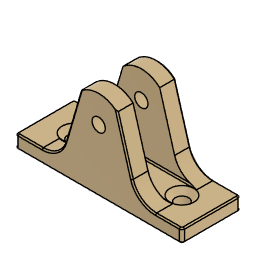
Trava toldo Regal v2 (Autodesk Fusion 360 design; units mm, degrees)
Autodesk Fusion 360 part; units mm, degrees
sketch "Sketch1" plane through (0, 0, 0) normal (0, 1, 0) x (1, 0, 0)
  line L0 (0, 0) -> (62.5, 0)
  line L1 (62.5, 0) -> (62.5, -5)
  line L2 (62.5, -5) -> (52.5, -5)
  arc A0 (52.5, -5) -> (43.75, -11.5668) centre (52.5, -14.1129) ccw
  line L3 (43.75, -11.5668) -> (38.15, -30.812)
  arc A1 (24.35, -30.812) -> (38.15, -30.812) centre (31.25, -23.3) ccw
  line L4 (24.35, -30.812) -> (18.75, -11.5668)
  arc A2 (18.75, -11.5668) -> (10, -5) centre (10, -14.1129) ccw
  line L5 (10, -5) -> (0, -5)
  line L6 (0, -5) -> (0, 0)
  circle A3 centre (31.25, -23.3) radius 2.5
  line L7 (24.35, -30.812) -> (38.15, -30.812) construction
  line L8 (31.25, -33.5) -> (31.25, -23.3) construction
  line L9 (10, -5) -> (52.5, -5)
  dimension "d1" = 13.8
  dimension "d2" = 7.7
  dimension "d3" = 5
  dimension "d5" = 5
  dimension "d8" = 62.5
  dimension "d29" = 33.5
  dimension "d30" = 25
  dimension "d31" = 10
  constraint coincident L0.start L6.end
  constraint horizontal L0
  constraint perpendicular L0 L1
  constraint perpendicular L1 L2
  constraint tangent L2 A0
  constraint tangent L4 A2
  constraint horizontal L5
  constraint perpendicular L0 L6
  constraint concentric A1 A3
  constraint horizontal L7
  constraint equal L3 L4
  constraint tangent A2 L5
  constraint tangent A0 L3
  constraint midpoint A1 L8.start
  constraint coincident A1.centre A3.centre
  constraint equal L2 L5
  constraint equal L1 L6
  constraint equal A0 A2
  measures "d1" distance of L3.end A1.start
  measures "d2" distance of A1 A3
  measures "d3" diameter of A3
  measures "d5" distance of L5.end L0.start
  measures "d8" distance of L0.start L0.end
  measures "d29" distance of L0 L8.start
  measures "d30" distance of A0.end L4.end
  measures "d31" distance of A2.end L5.end
extrude "Extrude1" add sketch "Sketch1" along normal blind 6
extrude "Extrude2" add sketch "Sketch1" against normal blind 10 contours L0 L1 L2 L5 L6 L9
extrude "Extrude3" add 1 faces at (31.3123, 6, 14.6469) along direction (0, -1, 0) blind 6 from surface at 16
fillet "Fillet1" radius 1 4 edges at (0, -16, 2.5) (62.5, -16, 2.5) (62.5, 6, 2.5) (0, 6, 2.5)
sketch "Sketch2" plane through (0, 0, 0) normal (0, 0, -1) x (1, 0, 0)
  arc A0 (0, -5) -> (1, -6) centre (1, -5) ccw
  line L0 (1, -6) -> (61.5, -6)
  arc A1 (61.5, -6) -> (62.5, -5) centre (61.5, -5) ccw
  line L1 (62.5, -5) -> (62.5, 15)
  arc A2 (62.5, 15) -> (61.5, 16) centre (61.5, 15) ccw
  line L2 (61.5, 16) -> (1, 16)
  arc A3 (1, 16) -> (0, 15) centre (1, 15) ccw
  line L3 (0, 15) -> (0, -5)
  line L4 (0, 5) -> (62.5, 5) construction
  circle A4 centre (11, 5) radius 2.5
  circle A5 centre (51.5, 5) radius 2.5
  line L5 (31.25, 5) -> (31.25, 16) construction
  dimension "d20" = 40.5
  dimension "d21" = 5
  constraint midpoint L3 L4.start
  constraint midpoint L1 L4.end
  constraint coincident L4 A4.centre
  constraint coincident L4 A5.centre
  constraint equal A4 A5
  constraint midpoint L4 L5.start
  constraint midpoint L2 L5.end
  constraint symmetric A4 A5 L5
  measures "d20" distance of A4.centre A5.centre
  measures "d21" diameter of A4
extrude "Extrude4" cut sketch "Sketch2" against normal blind 7 contours A4 | A5
chamfer "Chamfer1" distance 2 angle 45 2 edges at (8.6692, -4.096, 5) (49.1692, -4.096, 5)
chamfer "Chamfer2" distance 0.5 angle 45 27 edges at (40.95, 6, 21.1894) (47.03, 6, 6.8243) (57, 6, 5) (62.2071, 5.7071, 5) (62.5, -5, 5) (62.2071, -15.7071, 5) (57, -16, 5) (47.03, -16, 6.8243) (40.95, -16, 21.1894) (21.55, 6, 21.1894) (21.55, -16, 21.1894) (15.47, -16, 6.8243) (5.5, -16, 5) (0.2929, -15.7071, 5) (0, -5, 5) (0.2929, 5.7071, 5) (5.5, 6, 5) (15.47, 6, 6.8243) (31.25, 6, 33.5) (31.25, 6, 0) (0.2929, 5.7071, 0) (0, -5, 0) (0.2929, -15.7071, 0) (31.25, -16, 0) (62.2071, -15.7071, 0) (62.5, -5, 0) (62.2071, 5.7071, 0)
fillet "Fillet3" radius 0.5 2 edges at (31.25, -10, 5) (31.25, 0, 5)
